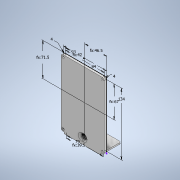
# Autodesk Inventor part: rear_case
Saved by Autodesk Inventor 2022.1 (Build 261234020, 234B)
## iProperties
Created: 2022-02-07
Part Number: rear_case
Material: Generic
Document SubType Name: Modeling
Designer: kee
Density: 1 g/cm^3
Appearance: Default
Mass: 80.2455 g
Surface Area: 378.529 cm^2
Volume: 80.2455 cm^3
Author: kee
Autodesk Inventor part; units mm, degrees
ref_plane "YZ Plane" through (0, 0, 0) normal (1, 0, 0) x (0, 1, 0)
ref_plane "XZ Plane" through (0, 0, 0) normal (0, 1, 0) x (-1, 0, 0)
ref_plane "XY Plane" through (0, 0, 0) normal (0, 0, 1) x (1, 0, 0)
sketch "Sketch3" plane through (0, 0, 0) normal (0, 0, 1) x (1, 0, 0)
  line L0 (42.5, 71.5) -> (-42.5, 71.5)
  line L1 (-46.5, 67.5) -> (-46.5, -67.5)
  line L2 (46.5, -67.5) -> (46.5, 67.5)
  line L3 (-42, 67) -> (42, 67) construction
  line L4 (42, 67) -> (42, -67) construction
  line L5 (42, -67) -> (-42, -67) construction
  line L6 (-42, -67) -> (-42, 67) construction
  arc A0 (-42.5, 71.5) -> (-46.5, 67.5) centre (-42.5, 67.5) ccw
  arc A1 (46.5, 67.5) -> (42.5, 71.5) centre (42.5, 67.5) ccw
  arc A2 (42.5, -71.5) -> (46.5, -67.5) centre (42.5, -67.5) ccw
  arc A3 (-46.5, -67.5) -> (-42.5, -71.5) centre (-42.5, -67.5) ccw
  line L7 (-39.5, -71.5) -> (-39.5, -74.9527)
  line L8 (-39.5, -74.9527) -> (39.5, -74.9527)
  line L9 (39.5, -74.9527) -> (39.5, -71.5)
  line L10 (-42.5, -71.5) -> (-39.5, -71.5)
  line L11 (39.5, -71.5) -> (42.5, -71.5)
  point P0 (0, 0)
  point P1 (46.5, 71.5)
  point P2 (-46.5, -71.5)
  point P3 (-46.5, 71.5)
  point P4 (46.5, -71.5)
  dimension "d7" = 93
  dimension "d9" = 46.5
  dimension "d10" = 71.5
  dimension "d11" = 84
  dimension "d12" = 134
  dimension "d13" = 42
  dimension "d14" = 67
  dimension "d15" = 4
  dimension "d16" = 4
  dimension "d17" = 79
  dimension "d18" = 39.5
  constraints: 24 end point, 10 tangent, 8 point on circle, 7 perpendicular, 6 point on line, 5 parallel, 4 centre point, 2 equal radius, 2 horizontal
  measures "d7" distance between parallel lines of L1 L2
  measures "d9" horizontal distance of point (0, 0) point (46.5, 71.5)
  measures "d10" vertical distance of point (-46.5, 71.5) point (0, 0)
  measures "d11" distance of L3.start L3.end
  measures "d12" distance of L3.end L4.end
  measures "d13" horizontal distance of point (0, 0) L3.start
  measures "d14" vertical distance of L3.end point (0, 0)
  measures "d15" radius of A0
  measures "d16" radius of A1
  measures "d17" distance of L7.end L8.end
  measures "d18" horizontal distance of point (0, 0) L7.end
extrude "Extrusion3" add sketch "Sketch3" along normal blind 5
sketch "Sketch4" plane through (0, 0, 0) normal (0, 0, -1) x (-1, 0, 0)
  line L0 (-39.642, -71.9527) -> (39.5, -71.9527)
  line L1 (39.5, -71.9527) -> (39.5, -74.9527)
  line L2 (39.5, -74.9527) -> (-39.5, -74.9527)
  line L3 (-39.5, -74.9527) -> (-39.5, -71.5)
  point P0 (0, 0)
  point P1 (-39.5, -71.9527)
  dimension "d46" = 3
  constraints: 8 end point, 2 coincident, 2 parallel, 1 horizontal, 1 perpendicular
  measures "d46" distance between parallel lines of L2 L0
extrude "Extrusion4" add sketch "Sketch4" along normal blind 38
fillet "Fillet1" radius 3 2 edges at (39.5, -73.4527, -38) (-39.5, -73.4527, -38)
sketch "Sketch5" plane through (0, 0, 5) normal (0, 0, 1) x (1, 0, 0)
  line L0 (-42, 67) -> (42, 67) construction
  line L1 (42, 67) -> (42, -67) construction
  line L2 (42, -67) -> (-42, -67) construction
  line L3 (-42, -67) -> (-42, 67) construction
  point P0 (0, 0)
  dimension "d22" = 134
  dimension "d23" = 84
  dimension "d24" = 42
  dimension "d25" = 67
  constraints: 8 end point, 4 coincident, 2 parallel, 1 horizontal, 1 perpendicular
  measures "d22" distance of L0.end L1.end
  measures "d23" distance of L1.end L2.end
  measures "d24" horizontal distance of L1.end point (0, 0)
  measures "d25" vertical distance of L0.end point (0, 0)
hole "Hole1" at (-42, 67, 5) at (42, 67, 5) at (-42, -67, 5) at (42, -67, 5) direction (0, 0, -1) diameter 3 end through all counterbore diameter 4.6 counterbore depth 2.5
sketch "Sketch6" plane through (0, 0, 5) normal (0, 0, 1) x (1, 0, 0)
  line L0 (39.5, -71.9527) -> (-39.5, -71.9527) projected
  line L1 (-1.5, -61.5) -> (1.5, -61.5) construction
  line L2 (-1.5, -66.5) -> (1.5, -66.5)
  line L3 (1.5, -56.5) -> (-1.5, -56.5)
  arc A0 (-1.5, -56.5) -> (-1.5, -66.5) centre (-1.5, -61.5) ccw
  arc A1 (1.5, -66.5) -> (1.5, -56.5) centre (1.5, -61.5) ccw
  point P0 (0, 0)
  point P1 (39.5, -71.5)
  point P2 (-39.5, -71.5)
  point P3 (0, -61.5)
  dimension "d35" = 10
  dimension "d36" = 10
  dimension "d37" = 3
  constraints: 8 end point, 4 point on circle, 4 tangent, 2 centre point, 1 horizontal, 1 horizontal alignment, 1 midpoint, 1 parallel, 1 vertical alignment
  measures "d35" diameter of A1
  measures "d36" vertical distance of point (39.5, -71.5) L1.end
  measures "d37" distance of L3.start L3.end
extrude "Extrusion5" cut sketch "Sketch6" against normal blind 5
sketch "Sketch7" plane through (0, 0, 0) normal (0, 0, -1) x (-1, 0, 0)
  line L0 (36.5, -71.9527) -> (-36.5, -71.9527) projected
  line L1 (-10, -71.9527) -> (10, -71.9527)
  line L2 (10, -71.9527) -> (10, -65.4527)
  line L3 (10, -65.4527) -> (-10, -65.4527)
  line L4 (-10, -65.4527) -> (-10, -71.9527)
  point P0 (0, 0)
  dimension "d40" = 6.5
  dimension "d41" = 20
  dimension "d42" = 10
  constraints: 8 end point, 2 parallel, 1 horizontal, 1 perpendicular, 1 point on line
  measures "d40" distance of L1.end L2.end
  measures "d41" distance of L2.end L3.end
  measures "d42" horizontal distance of point (0, 0) L3.end
extrude "Extrusion6" add sketch "Sketch7" along normal blind 20
sketch "Sketch8" plane through (0, 0, 0) normal (0, 0, -1) x (-1, 0, 0)
  line L0 (-30, 50) -> (30, 50) construction
  line L1 (30, 50) -> (30, -30) construction
  line L2 (30, -30) -> (-30, -30) construction
  line L3 (-30, -30) -> (-30, 50) construction
  circle A0 centre (-30, 50) radius 6
  circle A1 centre (30, 50) radius 6
  circle A2 centre (-30, -30) radius 6
  circle A3 centre (30, -30) radius 6
  point P0 (0, 0)
  dimension "d47" = 60
  dimension "d48" = 80
  dimension "d49" = 30
  dimension "d50" = 50
  dimension "d51" = 12
  dimension "d52" = 12
  dimension "d53" = 12
  dimension "d54" = 12
  constraints: 8 end point, 4 centre point, 4 coincident, 2 parallel, 1 horizontal, 1 perpendicular
  measures "d47" distance of L1.end L2.end
  measures "d48" distance between parallel lines of L0 L2
  measures "d49" horizontal distance of point (0, 0) L2.end
  measures "d50" vertical distance of L0.end point (0, 0)
  measures "d51" diameter of A0
  measures "d52" diameter of A1
  measures "d53" diameter of A2
  measures "d54" diameter of A3
chamfer "Chamfer1" distance 3 angle 45 4 edges at (0, -66.5, 5) (-6.5, -61.5, 5) (0, -56.5, 5) (6.5, -61.5, 5)
extrude "Extrusion7" add sketch "Sketch8" along normal blind 5
sketch "Sketch9" plane through (30, 50, -5) normal (0, 0, -1) x (-1, 0, 0)
  circle A0 centre (0, 0) radius 6 projected
  circle A1 centre (0, -80) radius 6 projected
  circle A2 centre (60, -80) radius 6 projected
  circle A3 centre (60, 0) radius 6 projected
  point P0 (30, -50)
  constraints: 4 coincident
hole "Hole2" at (30, 50, -5) at (-30, 50, -5) at (30, -30, -5) at (-30, -30, -5) direction (0, 0, 1) diameter 3 depth 4 tip angle 118
sketch "Sketch10" plane through (0, 0, 0) normal (0, 0, -1) x (-1, 0, 0)
  line L0 (-46.5, -42.9301) -> (46.5, -42.9301) construction
  line L1 (46.5, -42.9301) -> (46.5, -51.5) construction
  line L2 (46.5, -51.5) -> (-46.5, -51.5) construction
  line L3 (-46.5, -51.5) -> (-46.5, -42.9301) construction
  line L4 (-46.5, -67.5) -> (-46.5, 67.5) projected
  line L5 (46.5, 67.5) -> (46.5, -67.5) projected
  line L6 (-1.5, -56.5) -> (1.5, -56.5) projected
  spline S0 degree 2 poles (-25.231, -50.0404) (-25.231, -50.1305) (-25.2479, -50.2545) (-25.293, -50.3446) (-25.3493, -50.3841) (-25.3944, -50.3841) knots 0 0 0 1 2 3 4 4 4
  line L7 (-25.3944, -50.3841) -> (-28.0366, -50.3841)
  spline S1 degree 2 poles (-28.0366, -50.3841) (-28.138, -50.3841) (-28.3296, -50.2432) (-28.3296, -50.0629) knots 0 0 0 1 2 2 2
  line L8 (-28.3296, -50.0629) -> (-28.3296, -44.5305)
  spline S2 degree 2 poles (-28.3296, -44.5305) (-28.3296, -44.4967) (-28.2901, -44.4404) (-28.2, -44.4066) (-28.0423, -44.3841) (-27.9296, -44.3841) knots 0 0 0 1 2 3 4 4 4
  spline S3 degree 2 poles (-27.9296, -44.3841) (-27.8169, -44.3841) (-27.6648, -44.4066) (-27.5746, -44.4404) (-27.5352, -44.4967) (-27.5352, -44.5305) knots 0 0 0 1 2 3 4 4 4
  line L9 (-27.5352, -44.5305) -> (-27.5352, -49.6967)
  line L10 (-27.5352, -49.6967) -> (-25.3944, -49.6967)
  spline S4 degree 2 poles (-25.3944, -49.6967) (-25.3493, -49.6967) (-25.293, -49.7362) (-25.2479, -49.815) (-25.231, -49.9446) (-25.231, -50.0404) knots 0 0 0 1 2 3 4 4 4
  spline S5 degree 2 poles (-20.5831, -48.1474) (-20.5831, -48.6545) (-20.8479, -49.5108) (-21.3831, -50.1249) (-22.1775, -50.4742) (-22.707, -50.4742) knots 0 0 0 1 2 3 4 4 4
  spline S6 degree 2 poles (-22.707, -50.4742) (-23.2197, -50.4742) (-23.9803, -50.17) (-24.4873, -49.5897) (-24.7352, -48.7559) (-24.7352, -48.2263) knots 0 0 0 1 2 3 4 4 4
  spline S7 degree 2 poles (-24.7352, -48.2263) (-24.7352, -47.7193) (-24.4704, -46.8686) (-23.9408, -46.2488) (-23.1465, -45.9052) (-22.6169, -45.9052) knots 0 0 0 1 2 3 4 4 4
  spline S8 degree 2 poles (-22.6169, -45.9052) (-22.1042, -45.9052) (-21.3437, -46.2094) (-20.8366, -46.7897) (-20.5831, -47.6235) (-20.5831, -48.1474) knots 0 0 0 1 2 3 4 4 4
  spline S9 degree 2 poles (-21.3718, -48.1981) (-21.3718, -47.8601) (-21.4958, -47.2573) (-21.7887, -46.8066) (-22.2789, -46.5418) (-22.6451, -46.5418) knots 0 0 0 1 2 3 4 4 4
  spline S10 degree 2 poles (-22.6451, -46.5418) (-22.9887, -46.5418) (-23.4789, -46.7841) (-23.7944, -47.2235) (-23.9465, -47.8207) (-23.9465, -48.1756) knots 0 0 0 1 2 3 4 4 4
  spline S11 degree 2 poles (-23.9465, -48.1756) (-23.9465, -48.5193) (-23.8225, -49.1221) (-23.5296, -49.5672) (-23.0338, -49.8319) (-22.6676, -49.8319) knots 0 0 0 1 2 3 4 4 4
  spline S12 degree 2 poles (-22.6676, -49.8319) (-22.3296, -49.8319) (-21.8394, -49.5897) (-21.5183, -49.1559) (-21.3718, -48.5587) (-21.3718, -48.1981) knots 0 0 0 1 2 3 4 4 4
  spline S13 degree 2 poles (-15.9014, -50.2714) (-15.9014, -50.3052) (-15.9352, -50.3559) (-16.0141, -50.3953) (-16.1493, -50.4122) (-16.2451, -50.4122) knots 0 0 0 1 2 3 4 4 4
  spline S14 degree 2 poles (-16.2451, -50.4122) (-16.3521, -50.4122) (-16.4873, -50.3953) (-16.5662, -50.3559) (-16.5944, -50.3052) (-16.5944, -50.2714) knots 0 0 0 1 2 3 4 4 4
  line L11 (-16.5944, -50.2714) -> (-16.5944, -49.7193)
  spline S15 degree 2 poles (-16.5944, -49.7193) (-16.9493, -50.1136) (-17.6423, -50.4742) (-17.9972, -50.4742) knots 0 0 0 1 2 2 2
  spline S16 degree 2 poles (-17.9972, -50.4742) (-18.4141, -50.4742) (-18.9831, -50.1981) (-19.3324, -49.7193) (-19.4845, -49.0883) (-19.4845, -48.6376) knots 0 0 0 1 2 3 4 4 4
  line L12 (-19.4845, -48.6376) -> (-19.4845, -46.1136)
  spline S17 degree 2 poles (-19.4845, -46.1136) (-19.4845, -46.0798) (-19.4507, -46.0291) (-19.3606, -45.9841) (-19.2141, -45.9728) (-19.1014, -45.9728) knots 0 0 0 1 2 3 4 4 4
  spline S18 degree 2 poles (-19.1014, -45.9728) (-18.9887, -45.9728) (-18.8423, -45.9841) (-18.7577, -46.0291) (-18.7183, -46.0798) (-18.7183, -46.1136) knots 0 0 0 1 2 3 4 4 4
  line L13 (-18.7183, -46.1136) -> (-18.7183, -48.5362)
  spline S19 degree 2 poles (-18.7183, -48.5362) (-18.7183, -48.9024) (-18.6113, -49.3418) (-18.3972, -49.6517) (-18.0648, -49.8207) (-17.8394, -49.8207) knots 0 0 0 1 2 3 4 4 4
  spline S20 degree 2 poles (-17.8394, -49.8207) (-17.5521, -49.8207) (-16.9887, -49.415) (-16.6676, -49.0207) knots 0 0 0 1 2 2 2
  line L14 (-16.6676, -49.0207) -> (-16.6676, -46.1136)
  spline S21 degree 2 poles (-16.6676, -46.1136) (-16.6676, -46.0798) (-16.6338, -46.0291) (-16.5437, -45.9841) (-16.3972, -45.9728) (-16.2845, -45.9728) knots 0 0 0 1 2 3 4 4 4
  spline S22 degree 2 poles (-16.2845, -45.9728) (-16.1718, -45.9728) (-16.0254, -45.9841) (-15.9408, -46.0291) (-15.9014, -46.0798) (-15.9014, -46.1136) knots 0 0 0 1 2 3 4 4 4
  line L15 (-15.9014, -46.1136) -> (-15.9014, -50.2714)
  spline S23 degree 2 poles (-13.7324, -50.2714) (-13.7324, -50.3052) (-13.7718, -50.3559) (-13.8507, -50.3953) (-13.9972, -50.4122) (-14.1155, -50.4122) knots 0 0 0 1 2 3 4 4 4
  spline S24 degree 2 poles (-14.1155, -50.4122) (-14.2282, -50.4122) (-14.3746, -50.3953) (-14.4592, -50.3559) (-14.493, -50.3052) (-14.493, -50.2714) knots 0 0 0 1 2 3 4 4 4
  line L16 (-14.493, -50.2714) -> (-14.493, -46.1136)
  spline S25 degree 2 poles (-14.493, -46.1136) (-14.493, -46.0855) (-14.4592, -46.0291) (-14.3746, -45.9897) (-14.2282, -45.9728) (-14.1155, -45.9728) knots 0 0 0 1 2 3 4 4 4
  spline S26 degree 2 poles (-14.1155, -45.9728) (-13.9972, -45.9728) (-13.8507, -45.9897) (-13.7718, -46.0291) (-13.7324, -46.0855) (-13.7324, -46.1136) knots 0 0 0 1 2 3 4 4 4
  line L17 (-13.7324, -46.1136) -> (-13.7324, -50.2714)
  spline S27 degree 2 poles (-13.6423, -44.7108) (-13.6423, -44.9812) (-13.8451, -45.1728) (-14.1155, -45.1728) knots 0 0 0 1 2 2 2
  spline S28 degree 2 poles (-14.1155, -45.1728) (-14.3859, -45.1728) (-14.5831, -44.9812) (-14.5831, -44.7221) knots 0 0 0 1 2 2 2
  spline S29 degree 2 poles (-14.5831, -44.7221) (-14.5831, -44.4517) (-14.3803, -44.2601) (-14.1099, -44.2601) knots 0 0 0 1 2 2 2
  spline S30 degree 2 poles (-14.1099, -44.2601) (-13.8394, -44.2601) (-13.6423, -44.4517) (-13.6423, -44.7108) knots 0 0 0 1 2 2 2
  spline S31 degree 2 poles (-9.7155, -49.139) (-9.7155, -49.4601) (-9.9521, -49.9559) (-10.3859, -50.2995) (-10.9831, -50.4742) (-11.3437, -50.4742) knots 0 0 0 1 2 3 4 4 4
  spline S32 degree 2 poles (-11.3437, -50.4742) (-11.569, -50.4742) (-11.969, -50.4066) (-12.2845, -50.2995) (-12.5099, -50.1812) (-12.6113, -50.0911) (-12.6563, -49.9221) (-12.6563, -49.7812) knots 0 0 0 1 2 3 4 5 6 6 6
  spline S33 degree 2 poles (-12.6563, -49.7812) (-12.6563, -49.6911) (-12.6394, -49.5728) (-12.6113, -49.4995) (-12.5606, -49.4657) (-12.5268, -49.4657) knots 0 0 0 1 2 3 4 4 4
  spline S34 degree 2 poles (-12.5268, -49.4657) (-12.4761, -49.4657) (-12.2789, -49.5897) (-11.9859, -49.7418) (-11.5916, -49.8657) (-11.3324, -49.8657) knots 0 0 0 1 2 3 4 4 4
  spline S35 degree 2 poles (-11.3324, -49.8657) (-11.1408, -49.8657) (-10.8254, -49.7812) (-10.5944, -49.6179) (-10.4704, -49.37) (-10.4704, -49.201) knots 0 0 0 1 2 3 4 4 4
  spline S36 degree 2 poles (-10.4704, -49.201) (-10.4704, -49.0263) (-10.6507, -48.7841) (-10.9437, -48.5981) (-11.3155, -48.4573) (-11.7042, -48.2995) (-12.0817, -48.1024) (-12.3746, -47.815) (-12.5549, -47.415) (-12.5549, -47.139) knots 0 0 0 1 2 3 4 5 6 7 8 8 8
  spline S37 degree 2 poles (-12.5549, -47.139) (-12.5549, -46.8911) (-12.3634, -46.446) (-11.9859, -46.108) (-11.4225, -45.9052) (-11.0394, -45.9052) knots 0 0 0 1 2 3 4 4 4
  spline S38 degree 2 poles (-11.0394, -45.9052) (-10.8761, -45.9052) (-10.5437, -45.9615) (-10.2732, -46.046) (-10.0873, -46.1418) (-9.9916, -46.215) (-9.9577, -46.2714) (-9.9408, -46.339) (-9.9296, -46.4404) (-9.9296, -46.5136) knots 0 0 0 1 2 3 4 5 6 7 8 8 8
  spline S39 degree 2 poles (-9.9296, -46.5136) (-9.9296, -46.5925) (-9.9408, -46.7108) (-9.9746, -46.7841) (-10.0197, -46.8179) (-10.0479, -46.8179) knots 0 0 0 1 2 3 4 4 4
  spline S40 degree 2 poles (-10.0479, -46.8179) (-10.093, -46.8179) (-10.2507, -46.7165) (-10.4986, -46.5981) (-10.8366, -46.4967) (-11.0507, -46.4967) knots 0 0 0 1 2 3 4 4 4
  spline S41 degree 2 poles (-11.0507, -46.4967) (-11.2479, -46.4967) (-11.5408, -46.5869) (-11.7324, -46.7446) (-11.8282, -46.97) (-11.8282, -47.0995) knots 0 0 0 1 2 3 4 4 4
  spline S42 degree 2 poles (-11.8282, -47.0995) (-11.8282, -47.2798) (-11.6423, -47.5221) (-11.3493, -47.708) (-10.9662, -47.8545) (-10.5775, -48.0122) (-10.1944, -48.2038) (-9.8958, -48.4855) (-9.7155, -48.8686) (-9.7155, -49.139) knots 0 0 0 1 2 3 4 5 6 7 8 8 8
  spline S43 degree 2 poles (-5.4394, -50.0404) (-5.4394, -50.1305) (-5.4563, -50.2545) (-5.5014, -50.3446) (-5.5577, -50.3841) (-5.6028, -50.3841) knots 0 0 0 1 2 3 4 4 4
  line L18 (-5.6028, -50.3841) -> (-8.2451, -50.3841)
  spline S44 degree 2 poles (-8.2451, -50.3841) (-8.3465, -50.3841) (-8.538, -50.2432) (-8.538, -50.0629) knots 0 0 0 1 2 2 2
  line L19 (-8.538, -50.0629) -> (-8.538, -44.5305)
  spline S45 degree 2 poles (-8.538, -44.5305) (-8.538, -44.4967) (-8.4986, -44.4404) (-8.4085, -44.4066) (-8.2507, -44.3841) (-8.138, -44.3841) knots 0 0 0 1 2 3 4 4 4
  spline S46 degree 2 poles (-8.138, -44.3841) (-8.0254, -44.3841) (-7.8732, -44.4066) (-7.7831, -44.4404) (-7.7437, -44.4967) (-7.7437, -44.5305) knots 0 0 0 1 2 3 4 4 4
  line L20 (-7.7437, -44.5305) -> (-7.7437, -49.6967)
  line L21 (-7.7437, -49.6967) -> (-5.6028, -49.6967)
  spline S47 degree 2 poles (-5.6028, -49.6967) (-5.5577, -49.6967) (-5.5014, -49.7362) (-5.4563, -49.815) (-5.4394, -49.9446) (-5.4394, -50.0404) knots 0 0 0 1 2 3 4 4 4
  spline S48 degree 2 poles (-1.5296, -50.2714) (-1.5296, -50.3277) (-1.6028, -50.3841) (-1.7324, -50.4122) (-1.8563, -50.4122) knots 0 0 0 1 2 3 3 3
  spline S49 degree 2 poles (-1.8563, -50.4122) (-1.9746, -50.4122) (-2.1211, -50.3841) (-2.1831, -50.3277) (-2.1831, -50.2714) knots 0 0 0 1 2 3 3 3
  line L22 (-2.1831, -50.2714) -> (-2.1831, -49.8601)
  spline S50 degree 2 poles (-2.1831, -49.8601) (-2.4535, -50.1474) (-3.1239, -50.4742) (-3.4958, -50.4742) knots 0 0 0 1 2 2 2
  spline S51 degree 2 poles (-3.4958, -50.4742) (-3.8282, -50.4742) (-4.3577, -50.3052) (-4.7296, -49.9784) (-4.938, -49.5052) (-4.938, -49.2066) knots 0 0 0 1 2 3 4 4 4
  spline S52 degree 2 poles (-4.938, -49.2066) (-4.938, -48.8517) (-4.6507, -48.3334) (-4.1155, -47.9897) (-3.3437, -47.8207) (-2.8592, -47.8207) knots 0 0 0 1 2 3 4 4 4
  line L23 (-2.8592, -47.8207) -> (-2.2845, -47.8207)
  line L24 (-2.2845, -47.8207) -> (-2.2845, -47.4995)
  spline S53 degree 2 poles (-2.2845, -47.4995) (-2.2845, -47.2573) (-2.3859, -46.8911) (-2.6113, -46.6488) (-2.9718, -46.5249) (-3.2366, -46.5249) knots 0 0 0 1 2 3 4 4 4
  spline S54 degree 2 poles (-3.2366, -46.5249) (-3.5183, -46.5249) (-3.9634, -46.6601) (-4.3014, -46.8179) (-4.5268, -46.9531) (-4.5831, -46.9531) knots 0 0 0 1 2 3 4 4 4
  spline S55 degree 2 poles (-4.5831, -46.9531) (-4.6225, -46.9531) (-4.6732, -46.9136) (-4.7183, -46.8404) (-4.7352, -46.7277) (-4.7352, -46.6601) knots 0 0 0 1 2 3 4 4 4
  spline S56 degree 2 poles (-4.7352, -46.6601) (-4.7352, -46.5418) (-4.7014, -46.4066) (-4.5775, -46.2883) (-4.2732, -46.1249) (-3.8789, -45.9953) (-3.4056, -45.9052) (-3.169, -45.9052) knots 0 0 0 1 2 3 4 5 6 6 6
  spline S57 degree 2 poles (-3.169, -45.9052) (-2.7183, -45.9052) (-2.093, -46.108) (-1.7042, -46.5024) (-1.5296, -47.0826) (-1.5296, -47.4714) knots 0 0 0 1 2 3 4 4 4
  line L25 (-1.5296, -47.4714) -> (-1.5296, -50.2714)
  line L26 (-2.2845, -48.3728) -> (-2.938, -48.3728)
  spline S58 degree 2 poles (-2.938, -48.3728) (-3.2479, -48.3728) (-3.7099, -48.4798) (-4.0197, -48.6883) (-4.1606, -48.9812) (-4.1606, -49.1672) knots 0 0 0 1 2 3 4 4 4
  spline S59 degree 2 poles (-4.1606, -49.1672) (-4.1606, -49.4939) (-3.7493, -49.877) (-3.3775, -49.877) knots 0 0 0 1 2 2 2
  spline S60 degree 2 poles (-3.3775, -49.877) (-3.0789, -49.877) (-2.5662, -49.5728) (-2.2845, -49.2573) knots 0 0 0 1 2 2 2
  line L27 (-2.2845, -49.2573) -> (-2.2845, -48.3728)
  spline S61 degree 2 poles (3.693, -48.1362) (3.693, -48.677) (3.4563, -49.539) (3, -50.1531) (2.3352, -50.4742) (1.907, -50.4742) knots 0 0 0 1 2 3 4 4 4
  spline S62 degree 2 poles (1.907, -50.4742) (1.7099, -50.4742) (1.3718, -50.3953) (1.0507, -50.2207) (0.7239, -49.9503) (0.5437, -49.7643) knots 0 0 0 1 2 3 4 4 4
  line L28 (0.5437, -49.7643) -> (0.5437, -50.2714)
  spline S63 degree 2 poles (0.5437, -50.2714) (0.5437, -50.3052) (0.5099, -50.3615) (0.4254, -50.3953) (0.3014, -50.4122) (0.2056, -50.4122) knots 0 0 0 1 2 3 4 4 4
  spline S64 degree 2 poles (0.2056, -50.4122) (0.1155, -50.4122) (-0.0141, -50.3953) (-0.0986, -50.3615) (-0.1268, -50.3052) (-0.1268, -50.2714) knots 0 0 0 1 2 3 4 4 4
  line L29 (-0.1268, -50.2714) -> (-0.1268, -44.1024)
  spline S65 degree 2 poles (-0.1268, -44.1024) (-0.1268, -44.0686) (-0.093, -44.0122) (-0.0085, -43.9728) (0.138, -43.9559) (0.2507, -43.9559) knots 0 0 0 1 2 3 4 4 4
  spline S66 degree 2 poles (0.2507, -43.9559) (0.369, -43.9559) (0.5155, -43.9728) (0.5944, -44.0122) (0.6338, -44.0686) (0.6338, -44.1024) knots 0 0 0 1 2 3 4 4 4
  line L30 (0.6338, -44.1024) -> (0.6338, -46.5869)
  spline S67 degree 2 poles (0.6338, -46.5869) (0.8197, -46.401) (1.1634, -46.1418) (1.4958, -45.9784) (1.8282, -45.9052) (2.0141, -45.9052) knots 0 0 0 1 2 3 4 4 4
  spline S68 degree 2 poles (2.0141, -45.9052) (2.4648, -45.9052) (3.107, -46.2657) (3.507, -46.8686) (3.693, -47.6855) (3.693, -48.1362) knots 0 0 0 1 2 3 4 4 4
  spline S69 degree 2 poles (2.9042, -48.2263) (2.9042, -47.9052) (2.8085, -47.3024) (2.5662, -46.8404) (2.1662, -46.5587) (1.8676, -46.5587) knots 0 0 0 1 2 3 4 4 4
  spline S70 degree 2 poles (1.8676, -46.5587) (1.7211, -46.5587) (1.4338, -46.6432) (1.1352, -46.8348) (0.8141, -47.1446) (0.6338, -47.3756) knots 0 0 0 1 2 3 4 4 4
  line L31 (0.6338, -47.3756) -> (0.6338, -49.0319)
  spline S71 degree 2 poles (0.6338, -49.0319) (0.9493, -49.415) (1.5239, -49.8207) (1.8338, -49.8207) knots 0 0 0 1 2 2 2
  spline S72 degree 2 poles (1.8338, -49.8207) (2.1268, -49.8207) (2.5324, -49.5446) (2.7859, -49.0826) (2.9042, -48.5136) (2.9042, -48.2263) knots 0 0 0 1 2 3 4 4 4
  spline S73 degree 2 poles (7.4507, -49.139) (7.4507, -49.4601) (7.2141, -49.9559) (6.7803, -50.2995) (6.1831, -50.4742) (5.8225, -50.4742) knots 0 0 0 1 2 3 4 4 4
  spline S74 degree 2 poles (5.8225, -50.4742) (5.5972, -50.4742) (5.1972, -50.4066) (4.8817, -50.2995) (4.6563, -50.1812) (4.5549, -50.0911) (4.5099, -49.9221) (4.5099, -49.7812) knots 0 0 0 1 2 3 4 5 6 6 6
  spline S75 degree 2 poles (4.5099, -49.7812) (4.5099, -49.6911) (4.5268, -49.5728) (4.5549, -49.4995) (4.6056, -49.4657) (4.6394, -49.4657) knots 0 0 0 1 2 3 4 4 4
  spline S76 degree 2 poles (4.6394, -49.4657) (4.6901, -49.4657) (4.8873, -49.5897) (5.1803, -49.7418) (5.5746, -49.8657) (5.8338, -49.8657) knots 0 0 0 1 2 3 4 4 4
  spline S77 degree 2 poles (5.8338, -49.8657) (6.0254, -49.8657) (6.3408, -49.7812) (6.5718, -49.6179) (6.6958, -49.37) (6.6958, -49.201) knots 0 0 0 1 2 3 4 4 4
  spline S78 degree 2 poles (6.6958, -49.201) (6.6958, -49.0263) (6.5155, -48.7841) (6.2225, -48.5981) (5.8507, -48.4573) (5.462, -48.2995) (5.0845, -48.1024) (4.7915, -47.815) (4.6113, -47.415) (4.6113, -47.139) knots 0 0 0 1 2 3 4 5 6 7 8 8 8
  spline S79 degree 2 poles (4.6113, -47.139) (4.6113, -46.8911) (4.8028, -46.446) (5.1803, -46.108) (5.7437, -45.9052) (6.1268, -45.9052) knots 0 0 0 1 2 3 4 4 4
  spline S80 degree 2 poles (6.1268, -45.9052) (6.2901, -45.9052) (6.6225, -45.9615) (6.893, -46.046) (7.0789, -46.1418) (7.1746, -46.215) (7.2085, -46.2714) (7.2254, -46.339) (7.2366, -46.4404) (7.2366, -46.5136) knots 0 0 0 1 2 3 4 5 6 7 8 8 8
  spline S81 degree 2 poles (7.2366, -46.5136) (7.2366, -46.5925) (7.2254, -46.7108) (7.1915, -46.7841) (7.1465, -46.8179) (7.1183, -46.8179) knots 0 0 0 1 2 3 4 4 4
  spline S82 degree 2 poles (7.1183, -46.8179) (7.0732, -46.8179) (6.9155, -46.7165) (6.6676, -46.5981) (6.3296, -46.4967) (6.1155, -46.4967) knots 0 0 0 1 2 3 4 4 4
  spline S83 degree 2 poles (6.1155, -46.4967) (5.9183, -46.4967) (5.6254, -46.5869) (5.4338, -46.7446) (5.338, -46.97) (5.338, -47.0995) knots 0 0 0 1 2 3 4 4 4
  spline S84 degree 2 poles (5.338, -47.0995) (5.338, -47.2798) (5.5239, -47.5221) (5.8169, -47.708) (6.2, -47.8545) (6.5887, -48.0122) (6.9718, -48.2038) (7.2704, -48.4855) (7.4507, -48.8686) (7.4507, -49.139) knots 0 0 0 1 2 3 4 5 6 7 8 8 8
  spline S85 degree 2 poles (14.2338, -50.0404) (14.2338, -50.1249) (14.2113, -50.2545) (14.1718, -50.3446) (14.0986, -50.3841) (14.0592, -50.3841) knots 0 0 0 1 2 3 4 4 4
  line L32 (14.0592, -50.3841) -> (10.7577, -50.3841)
  spline S86 degree 2 poles (10.7577, -50.3841) (10.6901, -50.3841) (10.5944, -50.3503) (10.5268, -50.277) (10.493, -50.1362) (10.493, -50.0348) knots 0 0 0 1 2 3 4 4 4
  spline S87 degree 2 poles (10.493, -50.0348) (10.493, -49.9446) (10.5099, -49.8038) (10.5549, -49.6967) (10.6282, -49.5953) (10.6845, -49.5334) knots 0 0 0 1 2 3 4 4 4
  line L33 (10.6845, -49.5334) -> (11.8789, -48.3052)
  spline S88 degree 2 poles (11.8789, -48.3052) (12.2958, -47.8826) (12.7972, -47.2066) (13.0676, -46.6545) (13.1521, -46.2038) (13.1521, -46.001) knots 0 0 0 1 2 3 4 4 4
  spline S89 degree 2 poles (13.1521, -46.001) (13.1521, -45.8038) (13.0169, -45.4488) (12.7634, -45.1841) (12.3859, -45.0263) (12.138, -45.0263) knots 0 0 0 1 2 3 4 4 4
  spline S90 degree 2 poles (12.138, -45.0263) (11.8451, -45.0263) (11.3831, -45.1841) (11.0338, -45.3643) (10.8028, -45.5221) (10.7465, -45.5221) knots 0 0 0 1 2 3 4 4 4
  spline S91 degree 2 poles (10.7465, -45.5221) (10.7127, -45.5221) (10.6563, -45.4826) (10.6225, -45.4038) (10.6056, -45.2629) (10.6056, -45.1672) knots 0 0 0 1 2 3 4 4 4
  spline S92 degree 2 poles (10.6056, -45.1672) (10.6056, -45.0995) (10.6169, -44.9981) (10.6394, -44.9193) (10.6732, -44.8573) (10.7859, -44.7615) (11.0563, -44.5925) (11.4676, -44.4348) (11.9634, -44.3221) (12.2338, -44.3221) knots 0 0 0 1 2 3 4 5 6 7 8 8 8
  spline S93 degree 2 poles (12.2338, -44.3221) (12.6676, -44.3221) (13.3211, -44.5643) (13.7493, -44.9925) (13.9634, -45.5559) (13.9634, -45.8714) knots 0 0 0 1 2 3 4 4 4
  spline S94 degree 2 poles (13.9634, -45.8714) (13.9634, -46.1587) (13.862, -46.7277) (13.5352, -47.3869) (12.9155, -48.1925) (12.3972, -48.7221) knots 0 0 0 1 2 3 4 4 4
  line L34 (12.3972, -48.7221) -> (11.4507, -49.708)
  line L35 (11.4507, -49.708) -> (14.0535, -49.708)
  spline S95 degree 2 poles (14.0535, -49.708) (14.093, -49.708) (14.1606, -49.7474) (14.2113, -49.8319) (14.2338, -49.9559) (14.2338, -50.0404) knots 0 0 0 1 2 3 4 4 4
  spline S96 degree 2 poles (19.2197, -47.3869) (19.2197, -48.0742) (19.0056, -49.2066) (18.4986, -50.0235) (17.6873, -50.4742) (17.0901, -50.4742) knots 0 0 0 1 2 3 4 4 4
  spline S97 degree 2 poles (17.0901, -50.4742) (16.5324, -50.4742) (15.7606, -50.0742) (15.2873, -49.2911) (15.0901, -48.1531) (15.0901, -47.4094) knots 0 0 0 1 2 3 4 4 4
  spline S98 degree 2 poles (15.0901, -47.4094) (15.0901, -46.7277) (15.3099, -45.5897) (15.8113, -44.7728) (16.6225, -44.3221) (17.2141, -44.3221) knots 0 0 0 1 2 3 4 4 4
  spline S99 degree 2 poles (17.2141, -44.3221) (17.7775, -44.3221) (18.5493, -44.7221) (19.0225, -45.5052) (19.2197, -46.6432) (19.2197, -47.3869) knots 0 0 0 1 2 3 4 4 4
  spline S100 degree 2 poles (18.4085, -47.4376) (18.4085, -46.9925) (18.3465, -46.2826) (18.2169, -45.7362) (18.0197, -45.3474) (17.7437, -45.0883) (17.3887, -44.9756) (17.169, -44.9756) knots 0 0 0 1 2 3 4 5 6 6 6
  spline S101 degree 2 poles (17.169, -44.9756) (16.7746, -44.9756) (16.2845, -45.3474) (16.0028, -45.9897) (15.9014, -46.8573) (15.9014, -47.3587) knots 0 0 0 1 2 3 4 4 4
  spline S102 degree 2 poles (15.9014, -47.3587) (15.9014, -48.0235) (16.0423, -48.9643) (16.3408, -49.5503) (16.8085, -49.8207) (17.1408, -49.8207) knots 0 0 0 1 2 3 4 4 4
  spline S103 degree 2 poles (17.1408, -49.8207) (17.4, -49.8207) (17.7887, -49.6573) (18.0704, -49.3474) (18.2563, -48.9136) (18.369, -48.3841) (18.4085, -47.77) (18.4085, -47.4376) knots 0 0 0 1 2 3 4 5 6 6 6
  spline S104 degree 2 poles (23.8113, -50.0404) (23.8113, -50.1249) (23.7887, -50.2545) (23.7493, -50.3446) (23.6761, -50.3841) (23.6366, -50.3841) knots 0 0 0 1 2 3 4 4 4
  line L36 (23.6366, -50.3841) -> (20.3352, -50.3841)
  spline S105 degree 2 poles (20.3352, -50.3841) (20.2676, -50.3841) (20.1718, -50.3503) (20.1042, -50.277) (20.0704, -50.1362) (20.0704, -50.0348) knots 0 0 0 1 2 3 4 4 4
  spline S106 degree 2 poles (20.0704, -50.0348) (20.0704, -49.9446) (20.0873, -49.8038) (20.1324, -49.6967) (20.2056, -49.5953) (20.262, -49.5334) knots 0 0 0 1 2 3 4 4 4
  line L37 (20.262, -49.5334) -> (21.4563, -48.3052)
  spline S107 degree 2 poles (21.4563, -48.3052) (21.8732, -47.8826) (22.3746, -47.2066) (22.6451, -46.6545) (22.7296, -46.2038) (22.7296, -46.001) knots 0 0 0 1 2 3 4 4 4
  spline S108 degree 2 poles (22.7296, -46.001) (22.7296, -45.8038) (22.5944, -45.4488) (22.3408, -45.1841) (21.9634, -45.0263) (21.7155, -45.0263) knots 0 0 0 1 2 3 4 4 4
  spline S109 degree 2 poles (21.7155, -45.0263) (21.4225, -45.0263) (20.9606, -45.1841) (20.6113, -45.3643) (20.3803, -45.5221) (20.3239, -45.5221) knots 0 0 0 1 2 3 4 4 4
  spline S110 degree 2 poles (20.3239, -45.5221) (20.2901, -45.5221) (20.2338, -45.4826) (20.2, -45.4038) (20.1831, -45.2629) (20.1831, -45.1672) knots 0 0 0 1 2 3 4 4 4
  spline S111 degree 2 poles (20.1831, -45.1672) (20.1831, -45.0995) (20.1944, -44.9981) (20.2169, -44.9193) (20.2507, -44.8573) (20.3634, -44.7615) (20.6338, -44.5925) (21.0451, -44.4348) (21.5408, -44.3221) (21.8113, -44.3221) knots 0 0 0 1 2 3 4 5 6 7 8 8 8
  spline S112 degree 2 poles (21.8113, -44.3221) (22.2451, -44.3221) (22.8986, -44.5643) (23.3268, -44.9925) (23.5408, -45.5559) (23.5408, -45.8714) knots 0 0 0 1 2 3 4 4 4
  spline S113 degree 2 poles (23.5408, -45.8714) (23.5408, -46.1587) (23.4394, -46.7277) (23.1127, -47.3869) (22.493, -48.1925) (21.9746, -48.7221) knots 0 0 0 1 2 3 4 4 4
  line L38 (21.9746, -48.7221) -> (21.0282, -49.708)
  line L39 (21.0282, -49.708) -> (23.631, -49.708)
  spline S114 degree 2 poles (23.631, -49.708) (23.6704, -49.708) (23.738, -49.7474) (23.7887, -49.8319) (23.8113, -49.9559) (23.8113, -50.0404) knots 0 0 0 1 2 3 4 4 4
  spline S115 degree 2 poles (28.6, -50.0404) (28.6, -50.1249) (28.5775, -50.2545) (28.538, -50.3446) (28.4648, -50.3841) (28.4254, -50.3841) knots 0 0 0 1 2 3 4 4 4
  line L40 (28.4254, -50.3841) -> (25.1239, -50.3841)
  spline S116 degree 2 poles (25.1239, -50.3841) (25.0563, -50.3841) (24.9606, -50.3503) (24.893, -50.277) (24.8592, -50.1362) (24.8592, -50.0348) knots 0 0 0 1 2 3 4 4 4
  spline S117 degree 2 poles (24.8592, -50.0348) (24.8592, -49.9446) (24.8761, -49.8038) (24.9211, -49.6967) (24.9944, -49.5953) (25.0507, -49.5334) knots 0 0 0 1 2 3 4 4 4
  line L41 (25.0507, -49.5334) -> (26.2451, -48.3052)
  spline S118 degree 2 poles (26.2451, -48.3052) (26.662, -47.8826) (27.1634, -47.2066) (27.4338, -46.6545) (27.5183, -46.2038) (27.5183, -46.001) knots 0 0 0 1 2 3 4 4 4
  spline S119 degree 2 poles (27.5183, -46.001) (27.5183, -45.8038) (27.3831, -45.4488) (27.1296, -45.1841) (26.7521, -45.0263) (26.5042, -45.0263) knots 0 0 0 1 2 3 4 4 4
  spline S120 degree 2 poles (26.5042, -45.0263) (26.2113, -45.0263) (25.7493, -45.1841) (25.4, -45.3643) (25.169, -45.5221) (25.1127, -45.5221) knots 0 0 0 1 2 3 4 4 4
  spline S121 degree 2 poles (25.1127, -45.5221) (25.0789, -45.5221) (25.0225, -45.4826) (24.9887, -45.4038) (24.9718, -45.2629) (24.9718, -45.1672) knots 0 0 0 1 2 3 4 4 4
  spline S122 degree 2 poles (24.9718, -45.1672) (24.9718, -45.0995) (24.9831, -44.9981) (25.0056, -44.9193) (25.0394, -44.8573) (25.1521, -44.7615) (25.4225, -44.5925) (25.8338, -44.4348) (26.3296, -44.3221) (26.6, -44.3221) knots 0 0 0 1 2 3 4 5 6 7 8 8 8
  spline S123 degree 2 poles (26.6, -44.3221) (27.0338, -44.3221) (27.6873, -44.5643) (28.1155, -44.9925) (28.3296, -45.5559) (28.3296, -45.8714) knots 0 0 0 1 2 3 4 4 4
  spline S124 degree 2 poles (28.3296, -45.8714) (28.3296, -46.1587) (28.2282, -46.7277) (27.9014, -47.3869) (27.2817, -48.1925) (26.7634, -48.7221) knots 0 0 0 1 2 3 4 4 4
  line L42 (26.7634, -48.7221) -> (25.8169, -49.708)
  line L43 (25.8169, -49.708) -> (28.4197, -49.708)
  spline S125 degree 2 poles (28.4197, -49.708) (28.4592, -49.708) (28.5268, -49.7474) (28.5775, -49.8319) (28.6, -49.9559) (28.6, -50.0404) knots 0 0 0 1 2 3 4 4 4
  point P0 (0, 0)
  point P1 (0, -56.5)
  dimension "d64" = 5
  constraints: 2 point on line, 1 midpoint, 2 other
  measures "d64" vertical distance of point (0, -56.5) L1.end
emboss "Emboss1" sketch "Sketch10" operation cut depth 3 direction (0, 0, 1)
equation "\"d9\" = 0.5 * d7"
equation "\"d10\" = 0.5 * d8"
equation "\"d13\" = 0.5 * d11"
equation "\"d14\" = 0.5 * d12"
equation "\"d18\" = 0.5 * d17"
equation "\"d24\" = 0.5 * d23"
equation "\"d25\" = 0.5 * d22"
equation "\"d49\" = 0.5 * d47"
equation "\"d8\" = 143"
body "Solid2"
